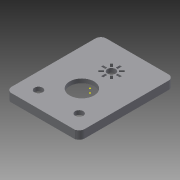
# Autodesk Inventor part: luz
Saved by Autodesk Inventor 2015 SP1 (Build 190203100, 203)
## iProperties
Created: 2015-07-05
Part Number: luz
Material: Genérico
Document SubType Name: Modeling
Designer: Javier
Density: 1 g/cm^3
Appearance: Valor por defecto
Author: Javier
Autodesk Inventor part; units mm, degrees
ref_plane "YZ Plane" through (0, 0, 0) normal (1, 0, 0) x (0, 1, 0)
ref_plane "XZ Plane" through (0, 0, 0) normal (0, 1, 0) x (-1, 0, 0)
ref_plane "XY Plane" through (0, 0, 0) normal (0, 0, 1) x (1, 0, 0)
sketch "Boceto1" plane through (0, 0, 0) normal (0, 0, 1) x (1, 0, 0)
  point P0 (0, 0)
sketch "Boceto2" plane through (0, 0, 0) normal (0, 0, 1) x (1, 0, 0)
  arc A0 (11.5, 13.5) -> (9.5, 15.5) centre (9.5, 13.5) ccw projected
  line L0 (9.5, 15.5) -> (-9.5, 15.5) projected
  arc A1 (-9.5, 15.5) -> (-11.5, 13.5) centre (-9.5, 13.5) ccw projected
  line L1 (-11.5, 13.5) -> (-11.5, -13.5) projected
  arc A2 (-11.5, -13.5) -> (-9.5, -15.5) centre (-9.5, -13.5) ccw projected
  line L2 (-9.5, -15.5) -> (9.5, -15.5) projected
  arc A3 (9.5, -15.5) -> (11.5, -13.5) centre (9.5, -13.5) ccw projected
  line L3 (11.5, -13.5) -> (11.5, 13.5) projected
  circle A4 centre (7.5, -11.5) radius 1.5 projected
  circle A5 centre (-7.5, -11.5) radius 1.5 projected
  line L4 (-4.5, 17.5) -> (-11.5, 17.5) projected
  arc A6 (-11.5, 17.5) -> (-13.5, 15.5) centre (-11.5, 15.5) ccw projected
  line L5 (-13.5, 15.5) -> (-13.5, -15.5) projected
  arc A7 (-13.5, -15.5) -> (-12.3012, -17.3325) centre (-11.5, -15.5) ccw projected
  arc A8 (-11.9943, -17.5) -> (-12.3012, -17.3325) centre (-13.1023, -19.165) ccw projected
  line L6 (11.9943, -17.5) -> (-11.9943, -17.5) projected
  arc A9 (12.3012, -17.3325) -> (11.9943, -17.5) centre (13.1023, -19.165) ccw projected
  arc A10 (12.3012, -17.3325) -> (13.5, -15.5) centre (11.5, -15.5) ccw projected
  line L7 (13.5, -15.5) -> (13.5, 15.5) projected
  arc A11 (13.5, 15.5) -> (11.5, 17.5) centre (11.5, 15.5) ccw projected
  line L8 (11.5, 17.5) -> (4.5, 17.5) projected
  line L9 (-4.5, 16.5) -> (-4.5, 17.5) projected
  line L10 (4.5, 17.5) -> (4.5, 16.5) projected
  line L11 (4.5, 16.5) -> (9.5, 16.5) projected
  arc A12 (12.5, 13.5) -> (9.5, 16.5) centre (9.5, 13.5) ccw projected
  line L12 (12.5, 13.5) -> (12.5, -13.5) projected
  arc A13 (9.5, -16.5) -> (12.5, -13.5) centre (9.5, -13.5) ccw projected
  line L13 (9.5, -16.5) -> (-9.5, -16.5) projected
  arc A14 (-12.5, -13.5) -> (-9.5, -16.5) centre (-9.5, -13.5) ccw projected
  line L14 (-12.5, -13.5) -> (-12.5, 13.5) projected
  arc A15 (-9.5, 16.5) -> (-12.5, 13.5) centre (-9.5, 13.5) ccw projected
  line L15 (-9.5, 16.5) -> (-4.5, 16.5) projected
  circle A16 centre (0, -6) radius 5.5 projected
  line L16 (-4.5, 15.5) -> (-4.5, 17.5)
  line L17 (4.5, 15.5) -> (4.5, 17.5)
  point P0 (0, 0)
  constraints: 4 end point, 2 point on line, 1 parallel, 1 vertical
extrude "Extrusión1" add sketch "Boceto2" along normal blind 1.5 contours A0 L0 L17 L11 A12 L12 A13 L13 A14 L14 A15 L15 L16 A1 L1 A2 L2 A3 L3 | L10 L8 A11 L7 A10 A9 L6 A8 A7 L5 A6 L4 L9 L15 A15 L14 A14 L13 A13 L12 A12 L11
sketch "Boceto3" plane through (0, 0, 1.5) normal (0, 0, 1) x (1, 0, 0)
  point P0 (0, 0)
lip "Labio1" kind lip height 1 width 1 edges at (11.5, 0, 0) (10.9142, -14.9142, 0) (0, -15.5, 0) (-10.9142, -14.9142, 0) (-11.5, 0, 0) (-10.9142, 14.9142, 0) (-7, 15.5, 0) (10.9142, 14.9142, 0) (7, 15.5, 0) guide face at (-12.8333, -4.5, 0)
sketch "Boceto4" plane through (0, 0, 1.5) normal (0, 0, 1) x (1, 0, 0)
  line L0 (-4.5, 17.5) -> (-11.5, 17.5) projected
  arc A0 (-11.5, 17.5) -> (-13.5, 15.5) centre (-11.5, 15.5) ccw projected
  line L1 (-13.5, 15.5) -> (-13.5, -15.5) projected
  arc A1 (-13.5, -15.5) -> (-12.3012, -17.3325) centre (-11.5, -15.5) ccw projected
  line L2 (-11.9943, -17.5) -> (11.9943, -17.5) projected
  arc A2 (12.3012, -17.3325) -> (13.5, -15.5) centre (11.5, -15.5) ccw projected
  line L3 (13.5, -15.5) -> (13.5, 15.5) projected
  arc A3 (13.5, 15.5) -> (11.5, 17.5) centre (11.5, 15.5) ccw projected
  line L4 (11.5, 17.5) -> (4.5, 17.5) projected
  line L5 (-4.5, 17.5) -> (4.5, 17.5)
  circle A4 centre (-7.5, -11.5) radius 1.5 projected
  circle A5 centre (7.5, -11.5) radius 1.5 projected
  line L6 (0, -15.5) -> (0, -3)
  circle A6 centre (0, -3) radius 4.5
  line L7 (12.3062, -17.3254) -> (11.9943, -17.5)
  arc A7 (12.3012, -17.3325) -> (11.9943, -17.5) centre (13.1023, -19.165) ccw projected
  line L8 (-12.3012, -17.3325) -> (-11.9943, -17.5)
  arc A8 (-11.9943, -17.5) -> (-12.3012, -17.3325) centre (-13.1023, -19.165) ccw projected
  dimension "d8" = 12.5
  dimension "d9" = 9
  constraints: 8 end point, 5 centre point, 1 coincident, 1 collinear, 1 vertical
  measures "d8" distance of L6.start L6.end
  measures "d9" diameter of A6
extrude "Extrusión2" add sketch "Boceto4" along normal blind 1.5 contours L5 L4 A3 L3 A2 A7 L2 A8 A1 L1 A0 L0
sketch "Boceto7" plane through (0, 0, 3) normal (0, 0, 1) x (1, 0, 0)
  circle A0 centre (0, -3) radius 4.5 projected
  circle A1 centre (7.5, -11.5) radius 1.5 projected
  circle A2 centre (-7.5, -11.5) radius 1.5 projected
  line L0 (11.5, 17.5) -> (-11.5, 17.5) projected
  arc A3 (-11.5, 17.5) -> (-13.5, 15.5) centre (-11.5, 15.5) ccw projected
  line L1 (-13.5, 15.5) -> (-13.5, -15.5) projected
  arc A4 (-13.5, -15.5) -> (-12.3012, -17.3325) centre (-11.5, -15.5) ccw projected
  line L2 (-11.9943, -17.5) -> (11.9943, -17.5) projected
  arc A5 (12.3012, -17.3325) -> (13.5, -15.5) centre (11.5, -15.5) ccw projected
  line L3 (13.5, -15.5) -> (13.5, 15.5) projected
  arc A6 (13.5, 15.5) -> (11.5, 17.5) centre (11.5, 15.5) ccw projected
  circle A7 centre (0, 7.9359) radius 1.5
  line L4 (-0.375, 11.3822) -> (0.375, 11.3822)
  line L5 (0.375, 11.3822) -> (0.375, 9.8822)
  line L6 (0.375, 9.8822) -> (-0.375, 9.8822)
  line L7 (-0.375, 9.8822) -> (-0.375, 11.3822)
  line L8 (-0.375, 11.3822) -> (0.375, 9.8822) construction
  line L9 (0.375, 11.3822) -> (-0.375, 9.8822) construction
  line L10 (-2.702, 10.1077) -> (-2.1717, 10.638)
  line L11 (-2.1717, 10.638) -> (-1.1111, 9.5773)
  line L12 (-1.1111, 9.5773) -> (-1.6414, 9.047)
  line L13 (-1.6414, 9.047) -> (-2.702, 10.1077)
  line L14 (-2.702, 10.1077) -> (-1.1111, 9.5773) construction
  line L15 (-2.1717, 10.638) -> (-1.6414, 9.047) construction
  line L16 (-3.4463, 7.5609) -> (-3.4463, 8.3109)
  line L17 (-3.4463, 8.3109) -> (-1.9463, 8.3109)
  line L18 (-1.9463, 8.3109) -> (-1.9463, 7.5609)
  line L19 (-1.9463, 7.5609) -> (-3.4463, 7.5609)
  line L20 (-3.4463, 7.5609) -> (-1.9463, 8.3109) construction
  line L21 (-3.4463, 8.3109) -> (-1.9463, 7.5609) construction
  line L22 (-2.1717, 5.2339) -> (-2.702, 5.7642)
  line L23 (-2.702, 5.7642) -> (-1.6414, 6.8249)
  line L24 (-1.6414, 6.8249) -> (-1.1111, 6.2946)
  line L25 (-1.1111, 6.2946) -> (-2.1717, 5.2339)
  line L26 (-2.1717, 5.2339) -> (-1.6414, 6.8249) construction
  line L27 (-2.702, 5.7642) -> (-1.1111, 6.2946) construction
  line L28 (0.375, 4.4897) -> (-0.375, 4.4897)
  line L29 (-0.375, 4.4897) -> (-0.375, 5.9897)
  line L30 (-0.375, 5.9897) -> (0.375, 5.9897)
  line L31 (0.375, 5.9897) -> (0.375, 4.4897)
  line L32 (0.375, 4.4897) -> (-0.375, 5.9897) construction
  line L33 (-0.375, 4.4897) -> (0.375, 5.9897) construction
  line L34 (2.702, 5.7642) -> (2.1717, 5.2339)
  line L35 (2.1717, 5.2339) -> (1.1111, 6.2946)
  line L36 (1.1111, 6.2946) -> (1.6414, 6.8249)
  line L37 (1.6414, 6.8249) -> (2.702, 5.7642)
  line L38 (2.702, 5.7642) -> (1.1111, 6.2946) construction
  line L39 (2.1717, 5.2339) -> (1.6414, 6.8249) construction
  line L40 (3.4463, 8.3109) -> (3.4463, 7.5609)
  line L41 (3.4463, 7.5609) -> (1.9463, 7.5609)
  line L42 (1.9463, 7.5609) -> (1.9463, 8.3109)
  line L43 (1.9463, 8.3109) -> (3.4463, 8.3109)
  line L44 (3.4463, 8.3109) -> (1.9463, 7.5609) construction
  line L45 (3.4463, 7.5609) -> (1.9463, 8.3109) construction
  line L46 (2.1717, 10.638) -> (2.702, 10.1077)
  line L47 (2.702, 10.1077) -> (1.6414, 9.047)
  line L48 (1.6414, 9.047) -> (1.1111, 9.5773)
  line L49 (1.1111, 9.5773) -> (2.1717, 10.638)
  line L50 (2.1717, 10.638) -> (1.6414, 9.047) construction
  line L51 (2.702, 10.1077) -> (1.1111, 9.5773) construction
  arc A8 (-11.9943, -17.5) -> (-12.3012, -17.3325) centre (-13.1023, -19.165) ccw projected
  arc A9 (12.3012, -17.3325) -> (11.9943, -17.5) centre (13.1023, -19.165) ccw projected
  point P0 (0, 10.6322)
  point P1 (-1.9066, 9.8425)
  point P2 (-2.6963, 7.9359)
  point P3 (-1.9066, 6.0294)
  point P4 (0, 5.2397)
  point P5 (1.9066, 6.0294)
  point P6 (2.6963, 7.9359)
  point P7 (1.9066, 9.8425)
  dimension "d38" = 3
  dimension "d39" = 0.75
  dimension "d40" = 1.5
  dimension "d43" = 360
  constraints: 96 end point, 16 midpoint, 2 parallel, 1 centre point, 1 horizontal, 1 perpendicular, 89 other
  measures "d38" diameter of A7
  measures "d39" distance of L5.end L6.end
  measures "d40" distance of L4.end L5.end
sketch "Boceto6" plane through (0, 0, 3) normal (0, 0, 1) x (1, 0, 0)
  arc A0 (-12.3012, -17.3325) -> (-11.9943, -17.5) centre (-13.1023, -19.165) ccw projected
  arc A1 (11.9943, -17.5) -> (12.3012, -17.3325) centre (13.1023, -19.165) ccw projected
  circle A2 centre (-13.1023, -19.165) radius 2
  circle A3 centre (13.1023, -19.165) radius 2
  point P0 (0, 0)
  constraints: 2 centre point, 2 coincident, 2 concentric
extrude "Extrusión4" cut sketch "Boceto6" against normal blind 10
extrude "Extrusión5" cut sketch "Boceto7" against normal blind 10 contours A7 | L4 L5 L6 L7 | L10 L11 L12 L13 | L16 L17 L18 L19 | L22 L23 L24 L25 | L28 L29 L30 L31 | L34 L35 L36 L37 | L40 L41 L42 L43 | L46 L47 L48 L49
